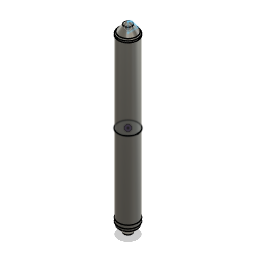
landing gear shaft v1 (Autodesk Fusion 360 design; units mm, degrees)
Autodesk Fusion 360 part; units mm, degrees
note: some values were not read from the file. Chosen so that the rebuilt part matches the saved one: which face or edge a step refers to.
sketch "Sketch1" plane through (0, 0, 0) normal (0, 1, 0) x (1, 0, 0)
  circle A0 centre (0, 0) radius 20
  dimension "d1" = 40
  constraint coincident A0.centre origin
  measures "d1" diameter of A0
extrude "Extrude1" add sketch "Sketch1" along normal blind 170 and the other way blind 170 makes body 1
sketch "Sketch2" plane through (0, 0, 0) normal (1, 0, 0) x (0, 0, -1)
  line L0 (20, 170) -> (0, 170)
  line L1 (0, 170) -> (0, 190)
  line L2 (20, 170) -> (8, 186)
  arc A0 (8, 186) -> (0, 190) centre (0, 180) ccw
  dimension "d6" = 20
  dimension "d7" = 20
  dimension "d8" = 10
  constraint horizontal L0
  constraint perpendicular L0 L1
  constraint coincident L1 A0.centre
  constraint tangent L2 A0
  measures "d6" distance of L0.end L1.end
  measures "d7" diameter of A0
  measures "d8" distance of L1.end A0.centre
revolve "Revolve1" add sketch "Sketch2" angle 360 about axis through (0, 0, 0) along (0, -1, 0) bodies 1
mirror "Mirror1" about plane through (0, 0, 0) normal (0, 1, 0) of "Extrude1", "Revolve1" makes body 2
fillet "Fillet1" radius 10 5 faces at (19.9751, -113.3333, 0.9969) (-2.57, 173.5556, -17.1417) (-1.4142, 187.0041, -6.9959) (-2.57, -173.5556, -17.1417) (-1.4142, -187.0041, -6.9959) on bodies 1 2
